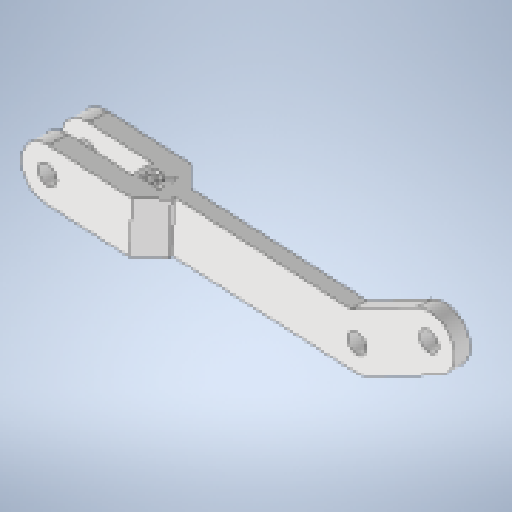
# Autodesk Inventor part: GripperShaftRight
Saved by Autodesk Inventor 2025.1 (Build 291241000, 241)
## iProperties
Created: 2026-05-06
Part Number: GripperShaftRight
Material: Generic
Document SubType Name: Modeling
Designer: User
Density: 1 g/cm^3
Appearance: Default
Author: User
## iProperties of the stored document GripperShaftRight_3DPrint.ipt
Created: 2026-05-06
Part Number: GripperShaftRight_3DPrint
Material: Generic
Document SubType Name: Modeling
Designer: User
Density: 1 g/cm^3
Appearance: Default
Author: User
Autodesk Inventor part; units mm, degrees
ref_plane "YZ Plane" through (0, 0, 0) normal (1, 0, 0) x (0, 1, 0)
ref_plane "XZ Plane" through (0, 0, 0) normal (0, 1, 0) x (-1, 0, 0)
ref_plane "XY Plane" through (0, 0, 0) normal (0, 0, 1) x (1, 0, 0)
sketch "Sketch1" plane through (0, 0, 0) normal (0, 0, 1) x (1, 0, 0)
  circle A0 centre (13.7198, 19.8458) radius 1.5 projected
  arc A1 (16.5482, 17.0174) -> (10.8914, 22.6743) centre (13.7198, 19.8458) ccw projected
  circle A2 centre (13.7198, 19.8458) radius 4
  line L0 (51.1915, 12.5598) -> (51.4214, 17.1106) projected
  line L1 (61.3785, 12.0451) -> (61.6084, 16.5959) projected
  line L2 (51.1915, 12.5598) -> (52.25, 33.5112)
  line L3 (13.7198, 19.8458) -> (51.4633, 17.9391)
  line L4 (13.518, 15.8509) -> (51.2615, 13.9442)
  line L5 (13.9216, 23.8407) -> (51.6651, 21.934)
  line L6 (48.1953, 12.7111) -> (47.9105, 7.0719) projected
  line L7 (48.2653, 14.0955) -> (48.6689, 22.0854)
  point P0 (0, 0)
  point P1 (10.8914, 22.6743)
  dimension "d0" = 8
  dimension "d1" = 4
  dimension "d2" = 4
  constraints: 10 end point, 3 point on line, 2 parallel, 2 perpendicular, 1 centre point, 1 coincident, 1 concentric
  measures "d0" diameter of A2
  measures "d1" distance between parallel lines of L3 L4
  measures "d2" distance between parallel lines of L3 L5
extrude "Extrusion1" add sketch "Sketch1" along normal blind 3 contours A1 A2 | A1 L5 L7 L3 | L3 L7 L4 A2 A1
sketch "Sketch2" plane through (0, 0, 0) normal (0, 0, -1) x (-1, 0, 0)
  line L0 (-51.4214, 17.1106) -> (-53.9776, 67.7102) projected
  line L1 (-61.6084, 16.5959) -> (-64.1646, 67.1956) projected
  line L2 (-48.6689, 22.0854) -> (-13.9216, 23.8407) projected
  line L3 (-13.518, 15.8509) -> (-48.2653, 14.0955) projected
  line L4 (-48.2653, 14.0955) -> (-48.6689, 22.0854) projected
  line L5 (-48.6689, 22.0854) -> (-48.2653, 14.0955)
  line L6 (-48.6689, 22.0854) -> (-48.2653, 14.0955)
  line L7 (-48.2653, 14.0955) -> (-23.2971, 15.3569)
  line L8 (-23.2971, 15.3569) -> (-23.7008, 23.3467)
  line L9 (-23.7008, 23.3467) -> (-48.6689, 22.0854)
  line L10 (-23.7008, 23.3467) -> (-23.2971, 15.3569)
  line L11 (-23.2971, 15.3569) -> (-61.4485, 13.4296)
  line L12 (-61.4485, 13.4296) -> (-61.8521, 21.4194)
  line L13 (-61.8521, 21.4194) -> (-23.7008, 23.3467)
  point P0 (0, 0)
  point P1 (-23.2971, 15.3569)
  point P2 (-23.7008, 23.3467)
  dimension "d5" = 25
  constraints: 18 end point, 7 equal length, 2 perpendicular
  measures "d5" distance of L7.end L3.end
extrude "Extrusion2" add sketch "Sketch2" along normal blind 3
sketch "Sketch3" plane through (0, 0, -3) normal (0, 0, -1) x (-1, 0, 0)
  line L0 (-48.2653, 14.0955) -> (-48.6689, 22.0854) projected
  line L1 (-48.6689, 22.0854) -> (-13.9216, 23.8407) projected
  arc A0 (-13.518, 15.8509) -> (-13.9216, 23.8407) centre (-13.7198, 19.8458) ccw projected
  line L2 (-13.518, 15.8509) -> (-48.2653, 14.0955) projected
  circle A1 centre (-13.7198, 19.8458) radius 1.5 projected
  line L3 (-23.2971, 15.3569) -> (-23.7008, 23.3467) projected
  line L4 (-26.2933, 15.2055) -> (-26.6969, 23.1953)
  point P0 (0, 0)
  dimension "d8" = 3
  constraints: 2 end point, 1 parallel
  measures "d8" distance between parallel lines of L3 L4
extrude "Extrusion3" add sketch "Sketch3" along normal blind 3.1 contours L4 L1 L3 L2 | L3 L1 A0 L2
sketch "Sketch4" plane through (0, 0, -3) normal (0, 0, 1) x (1, 0, 0)
  line L0 (23.2971, 15.3569) -> (23.7008, 23.3467) projected
  line L1 (13.9216, 23.8407) -> (23.7008, 23.3467) projected
  arc A0 (13.9216, 23.8407) -> (13.518, 15.8509) centre (13.7198, 19.8458) ccw projected
  line L2 (23.2971, 15.3569) -> (13.518, 15.8509) projected
  circle A1 centre (13.7198, 19.8458) radius 1.5 projected
  point P0 (0, 0)
extrude "Extrusion4" cut sketch "Sketch4" against normal blind 0.1
chamfer "Chamfer1" distance 3.1 angle 45 1 edges at (26.4951, 19.2004, -3)
sketch "Sketch5" plane through (0, 0, 3) normal (0, 0, 1) x (1, 0, 0)
  line L0 (48.2653, 14.0955) -> (48.6689, 22.0854) projected
  line L1 (48.6689, 22.0854) -> (13.9216, 23.8407) projected
  arc A0 (13.9216, 23.8407) -> (13.518, 15.8509) centre (13.7198, 19.8458) ccw projected
  line L2 (13.518, 15.8509) -> (48.2653, 14.0955) projected
  circle A1 centre (13.7198, 19.8458) radius 1.5 projected
  line L3 (26.6969, 23.1953) -> (26.2933, 15.2055) projected
  point P0 (0, 0)
extrude "Extrusion5" cut sketch "Sketch5" against normal blind 3 contours L2 L3 L1 L0
chamfer "Chamfer2" distance 3 angle 45 1 edges at (26.4951, 19.2004, 0)
sketch "Sketch6" plane through (0, 0, 0) normal (0, 0, 1) x (1, 0, 0)
  line L0 (29.2895, 15.0542) -> (29.6931, 23.044) projected
  line L1 (61.4485, 13.4296) -> (29.2895, 15.0542) projected
  line L2 (61.8521, 21.4194) -> (61.4485, 13.4296) projected
  line L3 (29.6931, 23.044) -> (61.8521, 21.4194) projected
  circle A0 centre (57.6554, 17.6263) radius 4
  circle A1 centre (57.6554, 17.6263) radius 1.5
  point P0 (0, 0)
  point P1 (57.8572, 21.6212)
  point P2 (61.6503, 17.4245)
  point P3 (57.4536, 13.6314)
  dimension "d21" = 3
  constraints: 3 tangent, 2 centre point, 1 coincident
  measures "d21" diameter of A1
extrude "Extrusion6" cut sketch "Sketch6" against normal blind 3 contours A0 L2 L1 | L3 L2 A0 | A1
sketch "Sketch7" plane through (13.9216, 23.8407, 3) normal (0.0504539, 0.9987264, 0) x (0.9987264, -0.0504539, 0)
  line L0 (34.7916, 3.3887) -> (37.7916, 3.3887) projected
  line L1 (43.9916, 6) -> (43.9916, 3) projected
  line L2 (15.8916, 6) -> (43.9916, 6) projected
  line L3 (12.7916, 9.1) -> (15.8916, 6) projected
  line L4 (0, 9.1) -> (12.7916, 9.1) projected
  line L5 (0, 6.1) -> (0, 9.1) projected
  line L6 (0, 6.1) -> (9.7916, 6.1) projected
  line L7 (9.7916, 3) -> (9.7916, 6.1) projected
  line L8 (9.7916, 3) -> (0, 3) projected
  line L9 (0, 3) -> (0, 0) projected
  line L10 (12.7916, 0) -> (0, 0) projected
  line L11 (15.7916, 3) -> (12.7916, 0) projected
  line L12 (15.7916, 3) -> (43.9916, 3) projected
  line L13 (34.7916, 3.5887) -> (37.7916, 3.5887)
  line L14 (34.7916, 3.5887) -> (49.1442, 3.5887)
  line L15 (49.1442, 3.5887) -> (49.1442, 2.3695)
  line L16 (49.1442, 2.3695) -> (34.7916, 2.3695)
  line L17 (34.7916, 2.3695) -> (34.7916, 3.5887)
  point P0 (-12.701, 3)
  dimension "d24" = 0.2
  constraints: 10 end point, 3 parallel, 1 horizontal, 1 perpendicular
  measures "d24" distance between parallel lines of L0 L13
extrude "Extrusion7" cut sketch "Sketch7" against normal through all contours L14 L15 L16 L17 L12 L1 | L1 L12 L17 L13 L14
sketch "Sketch8" plane through (0, 0, 0) normal (0, 0, 1) x (1, 0, 0)
  line L0 (48.2653, 14.0955) -> (48.6689, 22.0854) projected
  line L1 (29.6931, 23.044) -> (48.6689, 22.0854) projected
  line L2 (29.6931, 23.044) -> (48.2653, 14.0955)
  point P0 (0, 0)
  constraints: 2 end point
extrude "Extrusion8" cut sketch "Sketch8" against normal up to surface (0.5887 mm away)
sketch "Sketch9" plane through (13.9216, 23.8407, 3) normal (0.0504539, 0.9987264, 0) x (0.9987264, -0.0504539, 0)
  line L0 (10.584, 3.0196) -> (10.584, 6.0646) construction
  line L1 (10.584, 6.0646) -> (13.634, 6.0646) construction
  line L2 (13.634, 6.0646) -> (13.634, 3.0196) construction
  line L3 (13.634, 3.0196) -> (10.584, 3.0196) construction
  line L4 (13.634, 6.1536) -> (13.634, 5.2218)
  line L5 (13.634, 5.2218) -> (12.5143, 4.374)
  line L6 (12.5143, 4.374) -> (12.5143, 4.0972)
  line L7 (12.5143, 4.0972) -> (13.634, 4.0972)
  line L8 (13.634, 4.0972) -> (13.634, 3.3359)
  line L9 (13.634, 3.3359) -> (10.584, 3.3359)
  line L10 (10.584, 3.3359) -> (10.584, 4.5619)
  spline S0 degree 2 poles (10.584, 4.5619) (10.584, 4.8165) (10.6483, 5.1921) (10.7471, 5.3528) knots 0 0 0 1 2 2 2
  spline S1 degree 2 poles (10.7471, 5.3528) (10.8509, 5.5159) (11.1747, 5.7087) (11.4219, 5.7087) knots 0 0 0 1 2 2 2
  spline S2 degree 2 poles (11.4219, 5.7087) (11.7704, 5.7087) (12.2079, 5.3924) (12.3364, 5.1279) knots 0 0 0 1 2 2 2
  line L11 (12.3364, 5.1279) -> (13.634, 6.1536)
  spline S3 degree 2 poles (11.5183, 4.9227) (11.4021, 4.9227) (11.2365, 4.8338) (11.192, 4.7324) knots 0 0 0 1 2 2 2
  spline S4 degree 2 poles (11.192, 4.7324) (11.1624, 4.6607) (11.145, 4.4853) (11.145, 4.3543) knots 0 0 0 1 2 2 2
  line L12 (11.145, 4.3543) -> (11.145, 4.0972)
  line L13 (11.145, 4.0972) -> (11.9656, 4.0972)
  line L14 (11.9656, 4.0972) -> (11.9656, 4.3172)
  spline S5 degree 2 poles (11.9656, 4.3172) (11.9656, 4.4754) (11.9261, 4.7003) (11.8643, 4.7769) knots 0 0 0 1 2 2 2
  spline S6 degree 2 poles (11.8643, 4.7769) (11.805, 4.8511) (11.6468, 4.9227) (11.5183, 4.9227) knots 0 0 0 1 2 2 2
  point P0 (-12.701, 3)
  constraints: 2 other
emboss "Emboss1" sketch "Sketch9" operation cut depth 0.5 direction (-0.0504539, -0.9987264, 0)
sketch "Sketch10" plane through (0, 0, -3) normal (0, 0, -1) x (-1, 0, 0)
  circle A0 centre (-68.6887, 23.3886) radius 1.5 projected
  circle A1 centre (-57.6554, 17.6263) radius 1.5 projected
  line L0 (-29.3894, 15.0491) -> (-29.793, 23.0389) projected
  line L1 (-29.3894, 15.0491) -> (-57.4536, 13.6314) projected
  arc A2 (-59.5071, 14.0807) -> (-57.4536, 13.6314) centre (-57.6554, 17.6263) ccw projected
  line L2 (-59.5071, 14.0807) -> (-70.5404, 19.843) projected
  arc A3 (-66.837, 26.9342) -> (-70.5404, 19.843) centre (-68.6887, 23.3886) ccw projected
  line L3 (-66.837, 26.9342) -> (-56.7692, 21.6761) projected
  line L4 (-56.7692, 21.6761) -> (-29.793, 23.0389) projected
  arc A4 (-57.8572, 21.6212) -> (-57.4536, 13.6314) centre (-57.6554, 17.6263) ccw projected
  line L5 (-29.793, 23.0389) -> (-57.8572, 21.6212) projected
  point P0 (0, 0)
extrude "Extrusion9" add sketch "Sketch10" against normal up to surface (2.4113 mm away) contours L5 A4 L2 A3 L3
sketch "Sketch11" plane through (0, 0, 0) normal (0, 0, 1) x (1, 0, 0)
  line L0 (48.2653, 14.0955) -> (29.6931, 23.044) projected
  line L1 (29.2895, 15.0542) -> (29.6931, 23.044) projected
  line L2 (48.2653, 14.0955) -> (29.2895, 15.0542) projected
  point P0 (0, 0)
extrude "Extrusion10" cut sketch "Sketch11" against normal up to surface (0.5887 mm away)
body "Solid1"
